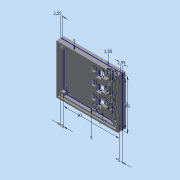
# Autodesk Inventor part: TopV2
Saved by Autodesk Inventor 2015 (Build 190159000, 159)
## iProperties
Created: 2014-12-30
Part Number: TopV2
Material: Generic
Document SubType Name: Modeling
Designer: Openlab
Density: 1 g/cm^3
Appearance: Default
Author: Openlab
Autodesk Inventor part; units mm, degrees
ref_plane "YZ Plane" through (0, 0, 0) normal (1, 0, 0) x (0, 1, 0)
ref_plane "XZ Plane" through (0, 0, 0) normal (0, 1, 0) x (-1, 0, 0)
ref_plane "XY Plane" through (0, 0, 0) normal (0, 0, 1) x (1, 0, 0)
sketch "Sketch1" plane through (0, 0, 0) normal (0, 1, 0) x (-1, 0, 0)
  line L0 (100, 0) -> (0, 0)
  line L1 (0, 0) -> (0, -80)
  line L2 (0, -80) -> (100, -80)
  line L3 (100, -80) -> (100, 0)
  line L4 (5, -5) -> (5, -75)
  line L5 (5, -75) -> (95, -75)
  line L6 (95, -75) -> (95, -5)
  line L7 (37.7, -8.55) -> (24.7, -8.55)
  line L8 (24.7, -8.55) -> (24.7, -21.55)
  line L9 (24.7, -21.55) -> (37.7, -21.55)
  line L10 (24.7, -48.55) -> (24.7, -61.55)
  line L11 (24.7, -61.55) -> (37.7, -61.55)
  line L12 (37.7, -48.55) -> (24.7, -48.55)
  line L13 (95, -75) -> (90, -75)
  line L14 (90, -75) -> (90, -70)
  line L15 (90, -70) -> (95, -70)
  line L16 (95, -70) -> (95, -75)
  line L17 (5, -5) -> (10, -5)
  line L18 (10, -5) -> (10, -10)
  line L19 (10, -10) -> (5, -10)
  line L20 (5, -10) -> (5, -5)
  line L21 (5, -75) -> (10, -75)
  line L22 (10, -75) -> (10, -70)
  line L23 (10, -70) -> (5, -70)
  line L24 (5, -70) -> (5, -75)
  line L25 (95, -5) -> (56.4, -5)
  line L26 (42.7, -65) -> (14.7, -65)
  line L27 (14.7, -5) -> (5, -5)
  line L28 (37.7, -56.3) -> (42.7, -56.3)
  line L29 (42.7, -53.8) -> (37.7, -53.8)
  line L30 (42.7, -36.3) -> (37.7, -36.3)
  line L31 (42.7, -33.8) -> (37.7, -33.8)
  line L32 (37.7, -16.3) -> (42.7, -16.3)
  line L33 (37.7, -13.8) -> (42.7, -13.8)
  line L34 (14.7, -57.3) -> (24.7, -57.3)
  line L35 (14.7, -52.8) -> (24.7, -52.8)
  line L36 (14.7, -37.3) -> (24.7, -37.3)
  line L37 (14.7, -32.8) -> (24.7, -32.8)
  line L38 (14.7, -17.3) -> (24.7, -17.3)
  line L39 (14.7, -12.8) -> (24.7, -12.8)
  line L40 (44.4, -5) -> (44.4, -65)
  line L41 (95, -5) -> (47.4, -5)
  line L42 (44.4, -5) -> (42.7, -5)
  line L43 (41.4, -75) -> (41.4, -72)
  line L44 (44.4, -5) -> (47.4, -5)
  line L45 (13, -5) -> (13, -72)
  line L46 (13, -72) -> (14.7, -72)
  line L47 (10, -70) -> (10, -5)
  line L48 (14.7, -72) -> (14.7, -75)
  line L49 (2.55, -77.45) -> (2.55, -2.55)
  line L50 (2.55, -2.55) -> (97.45, -2.55)
  line L51 (97.45, -2.55) -> (97.45, -77.45)
  line L52 (97.45, -77.45) -> (2.55, -77.45)
  line L53 (44.4, -65) -> (47.4, -65)
  line L54 (47.4, -75) -> (47.4, -72)
  line L55 (47.4, -65) -> (47.4, -5)
  line L56 (47.4, -72) -> (41.4, -72)
  line L57 (43.3668, -15.05) -> (15.15, -15.05) construction
  line L58 (37.7, -8.55) -> (37.7, -21.55)
  line L59 (45.3467, -35.05) -> (12.5232, -35.05) construction
  line L60 (14.8727, -55.05) -> (45.0542, -55.05) construction
  line L61 (42.7, -5) -> (42.7, -65)
  line L62 (37.7, -48.55) -> (37.7, -61.55)
  line L63 (37.7, -28.55) -> (24.7, -28.55)
  line L64 (24.7, -28.55) -> (24.7, -41.55)
  line L65 (24.7, -41.55) -> (37.7, -41.55)
  line L66 (37.7, -41.55) -> (37.7, -28.55)
  line L67 (90, -5) -> (90, -10)
  line L68 (90, -10) -> (95, -10)
  line L69 (14.7, -65) -> (14.7, -57.3)
  line L70 (14.7, -52.8) -> (14.7, -37.3)
  line L71 (14.7, -32.8) -> (14.7, -17.3)
  line L72 (14.7, -12.8) -> (14.7, -5)
  line L73 (16.2, -52.8) -> (16.2, -57.3)
  line L74 (16.2, -32.8) -> (16.2, -37.3)
  line L75 (16.2, -12.8) -> (16.2, -17.3)
  line L76 (42.7, -5) -> (14.7, -5)
  line L77 (14.7, -57.3) -> (14.7, -52.8)
  line L78 (14.7, -37.3) -> (14.7, -32.8)
  line L79 (14.7, -17.3) -> (14.7, -12.8)
  dimension "d0" = 5
  dimension "d1" = 5
  dimension "d2" = 5
  dimension "d4" = 13
  dimension "d5" = 70
  dimension "d8" = 5
  dimension "d9" = 5
  dimension "d10" = 5
  dimension "d11" = 5
  dimension "d12" = 5
  dimension "d13" = 5
  dimension "d16" = 90
  dimension "d18" = 80
  dimension "d24" = 2.5
  dimension "d27" = 4.5
  dimension "d28" = 4.5
  dimension "d29" = 4.5
  dimension "d31" = 60
  dimension "d34" = 3
  dimension "d36" = 2.55
  dimension "d37" = 2.55
  dimension "d38" = 2.55
  dimension "d39" = 2.55
  dimension "d40" = 3
  dimension "d41" = 6
  dimension "d42" = 3
  dimension "d43" = 13
  dimension "d44" = 12.5
  dimension "d45" = 20
  dimension "d46" = 20
  dimension "d47" = 13
  dimension "d48" = 5
  dimension "d49" = 1.7
  dimension "d51" = 13
  dimension "d52" = 2.5
  dimension "d53" = 2.5
  dimension "d54" = 5
  dimension "d62" = 3
  dimension "d63" = 1.7
  dimension "d64" = 10
  dimension "d65" = 8.5
  constraints: 160 end point, 36 point on line, 25 perpendicular, 21 parallel, 17 horizontal, 16 collinear, 5 vertical, 2 coincident, 9 other
  measures "d0" distance between parallel lines of L2 L5
  measures "d1" distance between parallel lines of L6 L3
  measures "d2" distance between parallel lines of L1 L4
  measures "d4" distance of L11.end L12.start
  measures "d5" distance of L4.start L4.end
  measures "d8" distance of L14.end L15.end
  measures "d9" distance of L13.end L14.end
  measures "d10" distance of L18.end L19.end
  measures "d11" distance of L17.end L18.end
  measures "d12" distance of L23.end L22.end
  measures "d13" distance of L22.end L21.end
  measures "d16" distance of L4.end L5.end
  measures "d18" distance between parallel lines of L0 L2
  measures "d24" distance between parallel lines of L31 L30
  measures "d27" distance between parallel lines of L39 L38
  measures "d28" distance between parallel lines of L37 L36
  measures "d29" distance between parallel lines of L34 L35
  measures "d31" distance of L26.end L27.start
  measures "d34" distance of L43.start L43.end
  measures "d36" distance between parallel lines of L1 L49
  measures "d37" distance between parallel lines of L0 L50
  measures "d38" distance between parallel lines of L2 L52
  measures "d39" distance between parallel lines of L3 L51
  measures "d40" distance of L40.end L53.end
  measures "d41" distance of L54.end L43.end
  measures "d42" distance of L46.end L48.end
  measures "d43" distance between parallel lines of L9 L7
  measures "d44" distance between parallel lines of L57 L50
  measures "d45" distance between parallel lines of L59 L57
  measures "d46" distance between parallel lines of L60 L59
  measures "d47" distance between parallel lines of L10 L62
  measures "d48" distance between parallel lines of L62 L61
  measures "d49" distance between parallel lines of L61 L40
  measures "d51" distance between parallel lines of L65 L63
  measures "d52" distance between parallel lines of L32 L33
  measures "d53" distance between parallel lines of L28 L29
  measures "d54" distance between parallel lines of L0 L25
  measures "d62" distance between parallel lines of L47 L45
  measures "d63" distance between parallel lines of L45 L72
  measures "d64" distance between parallel lines of L72 L8
  measures "d65" distance between parallel lines of L8 L75
extrude "Extrusion4" add sketch "Sketch1" against normal blind 5 contours L17 L18 L19 L4 | L23 L22 L5 L4 | L76 L61 L33 L58 L7 L8 L39 L72 | L38 L8 L9 L58 L32 L61 L31 L66 L63 L64 L37 L71 | L36 L64 L65 L66 L30 L61 L29 L62 L12 L10 L35 L70 | L14 L15 L6 L5 | L25 L6 L68 L67 | L34 L10 L11 L62 L28 L61 L26 L69 | L49 L50 L51 L52
extrude "Extrusion5" add sketch "Sketch1" against normal blind 7.5 contours L61 L32 L58 L33 | L61 L30 L66 L31 | L61 L28 L62 L29
extrude "Extrusion6" add sketch "Sketch1" against normal blind 2.5 contours L27 L45 L46 L48 L5 L22 L47 L18 | L44 L55 L53 L40 | L43 L56 L54 L5
extrude "Extrusion7" add sketch "Sketch1" against normal blind 10 contours L39 L8 L38 L75 | L37 L64 L36 L74 | L35 L10 L34 L73
extrude "Extrusion8" add sketch "Sketch1" along normal blind 3 contours L76 L61 L33 L58 L7 L8 L39 L72 | L39 L75 L38 L79 | L39 L8 L38 L75 | L38 L8 L9 L58 L32 L61 L31 L66 L63 L64 L37 L71 | L61 L32 L58 L33 | L37 L74 L36 L78 | L37 L64 L36 L74 | L36 L64 L65 L66 L30 L61 L29 L62 L12 L10 L35 L70 | L61 L30 L66 L31 | L35 L73 L34 L77 | L35 L10 L34 L73 | L34 L10 L11 L62 L28 L61 L26 L69 | L61 L28 L62 L29
extrude "Extrusion9" add sketch "Sketch1" along normal blind 5 contours L3 L2 L1 L0 | L17 L18 L19 L4 | L19 L47 L23 L4 | L27 L45 L46 L48 L5 L22 L47 L18 | L23 L22 L5 L4 | L27 L72 L79 L71 L78 L70 L77 L69 L26 L61 L42 L40 L53 L55 L41 L25 L67 L68 L6 L15 L14 L5 L54 L56 L43 L48 L46 L45 | L44 L55 L53 L40 | L43 L56 L54 L5 | L14 L15 L6 L5 | L25 L6 L68 L67 | L49 L50 L51 L52
fillet "Fillet1" radius 2 4 edges at (-28.7, 0, -65) (-45.9, 0, -65) (-47.4, 0, -35) (-10, 0, -40)
extrude "Extrusion10" add sketch "Sketch1" against normal blind 7.5 contours L3 L2 L1 L0
sketch "Sketch2" plane through (0, 5, 0) normal (0, 1, 0) x (1, 0, 0)
  line L0 (-100, 80) -> (-100, 0) projected
  line L1 (0, 80) -> (-100, 80) projected
  point P0 (0, 0)
  point P1 (-6, 6)
  point P2 (-94, 74)
  point P3 (-94, 6)
  point P4 (-6, 74)
  dimension "d81" = 6
  dimension "d82" = 6
  dimension "d83" = 6
  dimension "d84" = 6
  constraints: 2 horizontal alignment, 2 vertical alignment
  measures "d81" horizontal distance of point (0, 0) point (-6, 6)
  measures "d82" horizontal distance of point (0, 0) point (-6, 6)
  measures "d83" distance from line of L0 point (-94, 74)
  measures "d84" distance from line of L1 point (-94, 74)
hole "Hole1" at (-6, 5, -6) at (-6, 5, -74) at (-94, 5, -74) at (-94, 5, -6) direction (0, -1, 0) diameter 4 end through all counterbore diameter 6 counterbore depth 3
body "Solid2"
